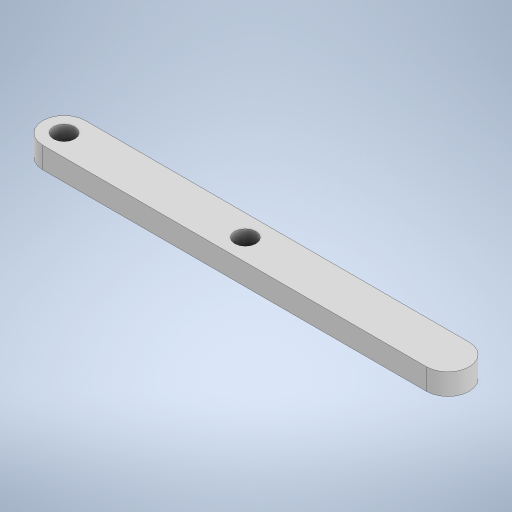
# Autodesk Inventor part: Hebel
Saved by Autodesk Inventor 2024 (Build 280153000, 153)
## iProperties
Created: 2023-08-23
Part Number: Hebel
Material: Generisch
Document SubType Name: Modeling
Designer: rapp
Density: 1 g/cm^3
Appearance: Vorgabe
Author: rapp
Autodesk Inventor part; units mm, degrees
ref_plane "YZ Plane" through (0, 0, 0) normal (1, 0, 0) x (0, 1, 0)
ref_plane "XZ Plane" through (0, 0, 0) normal (0, 1, 0) x (-1, 0, 0)
ref_plane "XY Plane" through (0, 0, 0) normal (0, 0, 1) x (1, 0, 0)
sketch "Skizze1" plane through (0, 0, 0) normal (0, 0, 1) x (1, 0, 0)
  line L0 (-25, 0) -> (115, 0) projected
  line L1 (0, -7) -> (0, 7) projected
  line L2 (0, 0) -> (90, 0) construction
  line L3 (0, -5) -> (90, -5)
  line L4 (90, 5) -> (0, 5)
  arc A0 (0, 5) -> (0, -5) centre (0, 0) ccw
  arc A1 (90, -5) -> (90, 5) centre (90, 0) ccw
  point P0 (45, 0)
  dimension "d0" = 90
  dimension "d1" = 10
  constraints: 8 end point, 4 point on circle, 4 tangent, 2 centre point, 1 midpoint, 1 parallel, 1 point on line
  measures "d0" distance of L2.start L2.end
  measures "d1" diameter of A1
extrude "Extrusion1" add sketch "Skizze1" along normal blind 5
sketch "Skizze2" plane through (0, 0, 5) normal (0, 0, 1) x (1, 0, 0)
  point P0 (0, 0)
  point P1 (0, 0)
  constraints: 1 coincident
hole "Bohrung1" at (0, 0, 5) direction (0, 0, -1) diameter 5 end through all
sketch "Skizze3" plane through (0, 0, 5) normal (0, 0, 1) x (1, 0, 0)
  point P0 (0, 0)
  point P1 (42.5, 0)
  dimension "d11" = 42.5
  measures "d11" distance of point (42.5, 0) point (0, 0)
hole "Bohrung2" at (42.5, 0, 5) direction (0, 0, -1) diameter 5 end through all
